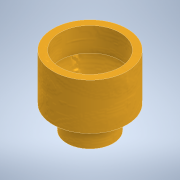
# Autodesk Inventor part: bottom injector
Saved by Autodesk Inventor 2021 (Build 250183000, 183)
## iProperties
Created: 2021-07-21
Part Number: bottom injector
Material: Brass, Soft Yellow, Welded
Document SubType Name: Modeling
Designer: samlo
Density: 8.5 g/cm^3
Appearance: Weld - Brass
Author: samlo
Autodesk Inventor part; units mm, degrees
ref_plane "YZ Plane" through (0, 0, 0) normal (1, 0, 0) x (0, 1, 0)
ref_plane "XZ Plane" through (0, 0, 0) normal (0, 1, 0) x (-1, 0, 0)
ref_plane "XY Plane" through (0, 0, 0) normal (0, 0, 1) x (1, 0, 0)
sketch "Sketch1" plane through (0, 0, 0) normal (0, 0, 1) x (1, 0, 0)
  line L0 (4, 0) -> (4, 5.5)
  line L1 (4, 5.5) -> (6.5, 9.8301)
  line L2 (6.5, 9.8301) -> (6.5, 15)
  line L3 (6.5, 15) -> (8, 15)
  line L4 (8, 15) -> (8, 5)
  line L5 (8, 5) -> (5, 5)
  line L6 (5, 5) -> (5, 0)
  line L7 (5, 0) -> (4, 0)
  line L8 (0, -3) -> (0, 18) projected
  point P0 (0, 0)
  dimension "d0" = 6.5
  dimension "d1" = 15
  dimension "d2" = 1.5
  dimension "d3" = 4
  dimension "d4" = 5
  dimension "d5" = 10
  dimension "d6" = 60
  dimension "d7" = 5.5
  dimension "d8" = 3
  constraints: 16 end point, 5 perpendicular, 1 parallel, 1 vertical
  measures "d0" distance from line of L2 point (0, 0)
  measures "d1" vertical distance of L0.start L2.end
  measures "d2" distance of L2.end L3.end
  measures "d3" distance of L0.start point (0, 0)
  measures "d4" distance of L6.end point (0, 0)
  measures "d5" distance of L3.end L4.end
  measures "d6" angle of L7 L1
  measures "d7" distance of L0.start L0.end
  measures "d8" distance of L4.end L5.end
revolve "Revolution1" add sketch "Sketch1" angle 360 about axis through (0, -10, 0) along (0, 1, 0)
body "Solid1"
